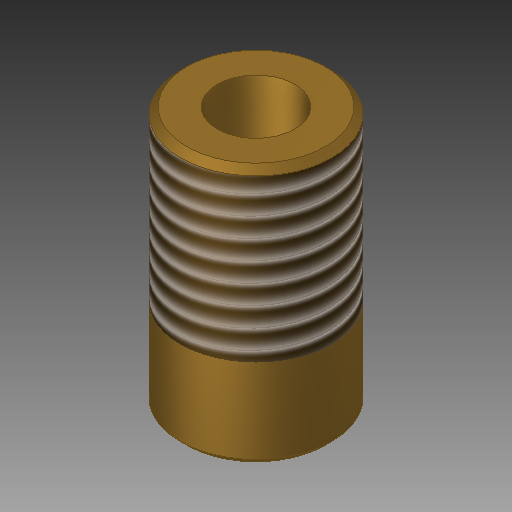
# Autodesk Inventor part: Schneckenwelle
Saved by Autodesk Inventor 2019 (Build 230136000, 136)
## iProperties
Created: 2021-11-05
Part Number: Schneckenwelle
Material: Messing, weicher Gelbton
Document SubType Name: Modeling
Designer: Bergi
Density: 8.47 g/cm^3
Appearance: Messing - satiniert
Mass: 13.3474 g
Surface Area: 12.4842 cm^2
Volume: 1.57585 cm^3
Author: Bergi
Autodesk Inventor part; units mm, degrees
ref_plane "YZ Plane" through (0, 0, 0) normal (1, 0, 0) x (0, 1, 0)
ref_plane "XZ Plane" through (0, 0, 0) normal (0, 1, 0) x (-1, 0, 0)
ref_plane "XY Plane" through (0, 0, 0) normal (0, 0, 1) x (1, 0, 0)
sketch "Skizze1" plane through (0, 0, 0) normal (0, 1, 0) x (-1, 0, 0)
  circle A0 centre (0, 0) radius 5.85
  dimension "d0" = 11.7
  constraints: 1 centre point, 1 coincident
  measures "d0" diameter of A0
extrude "Extrusion1" add sketch "Skizze1" along normal blind 20
thread "Gewinde1" size "TR8x1.5" class "7e" standard "ISO Metric Trapezoidal Threads" length 13
sketch "Skizze3" plane through (0, 0, 0) normal (0, -1, 0) x (1, 0, 0)
  circle A0 centre (0, 0) radius 3
  dimension "d5" = 6
  constraints: 1 centre point, 1 coincident
  measures "d5" diameter of A0
extrude "Extrusion2" cut sketch "Skizze3" against normal through all
chamfer "Fase1" distance 0.5 angle 45 2 edges at (5.85, 20, 0) (5.85, 0, 0)
